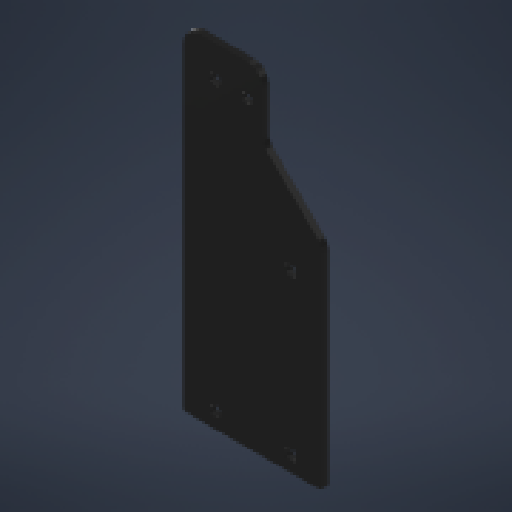
# Autodesk Inventor part: funnelFront
Saved by Autodesk Inventor 2025.2 (Build 292293000, 293)
## iProperties
Created: 2025-11-17
Part Number: funnelFront
Material: white pla
Document SubType Name: Modeling
Designer: cloudy
Density: 1 g/cm^3
Appearance: Smooth - Black
Author: cloudy
Autodesk Inventor part; units mm, degrees
ref_plane "YZ Plane" through (0, 0, 0) normal (1, 0, 0) x (0, 1, 0)
ref_plane "XZ Plane" through (0, 0, 0) normal (0, 1, 0) x (-1, 0, 0)
ref_plane "XY Plane" through (0, 0, 0) normal (0, 0, 1) x (1, 0, 0)
sketch "Sketch1" plane through (0, 0, 0) normal (0, 0, 1) x (1, 0, 0)
  circle A0 centre (-6.35, 171.45) radius 2.1844 projected
  circle A1 centre (6.35, 171.45) radius 2.1844 projected
  circle A2 centre (23.8125, 120.65) radius 2.1844 projected
  circle A3 centre (23.8125, 57.15) radius 2.1844 projected
  circle A4 centre (-6.35, 57.15) radius 2.1844 projected
  line L0 (-19.05, 50.8) -> (36.5125, 50.8)
  line L1 (36.5125, 50.8) -> (36.5125, 134.9375)
  line L2 (12.7, 184.15) -> (-19.05, 184.15)
  line L3 (-19.05, 184.15) -> (-19.05, 50.8)
  line L4 (12.7, 184.15) -> (12.7, 158.75)
  line L5 (12.7, 158.75) -> (36.5125, 134.9375)
  point P0 (0, 0)
  dimension "d0" = 12.7
  dimension "d2" = 12.7
  dimension "d3" = 6.35
  dimension "d4" = 12.7
  dimension "d15" = 25.4
  dimension "d16" = 31.75
  dimension "d17" = 135
  constraints: 12 end point, 3 vertical, 2 horizontal
  measures "d0" distance from line of L2 A1.centre
  measures "d2" distance from line of L3 A0.centre
  measures "d3" distance from line of L0 A4.centre
  measures "d4" distance from line of L1 A3.centre
  measures "d15" distance of L2.start L4.end
  measures "d16" distance between parallel lines of L3 L4
  measures "d17" angle of L4 L5
extrude "Extrusion1" add sketch "Sketch1" along normal blind 2.54
fillet "Fillet1" radius 6.35 4 edges at (-19.05, 184.15, 1.27) (12.7, 184.15, 1.27) (12.7, 158.75, 1.27) (36.5125, 134.9375, 1.27)
chamfer "Chamfer1" distance 0.7937 angle 45 2 edges at (36.5125, 50.8, 1.27) (-19.05, 50.8, 1.27)
body "Solid1"
